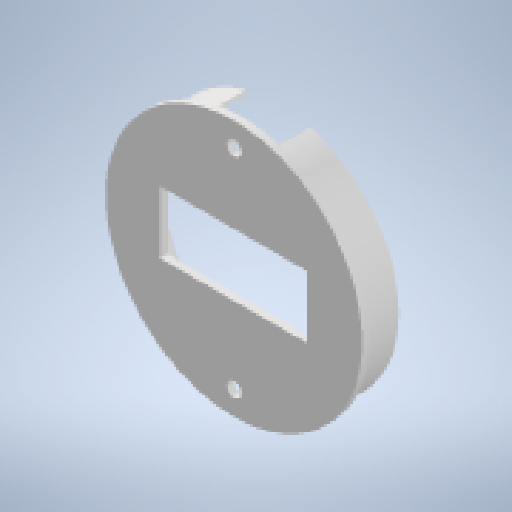
# Autodesk Inventor part: lid2
Saved by Autodesk Inventor 2025.3 (Build 293356000, 356)
## iProperties
Created: 2025-04-21
Part Number: lid2
Material: Generic
Document SubType Name: Modeling
Designer: Owner
Density: 1 g/cm^3
Appearance: Default
Author: Owner
Autodesk Inventor part; units mm, degrees
ref_plane "YZ Plane" through (0, 0, 0) normal (1, 0, 0) x (0, 1, 0)
ref_plane "XZ Plane" through (0, 0, 0) normal (0, 1, 0) x (-1, 0, 0)
ref_plane "XY Plane" through (0, 0, 0) normal (0, 0, 1) x (1, 0, 0)
sketch "Sketch1" plane through (0, 0, 0) normal (0, 0, 1) x (1, 0, 0)
  arc A0 (8.8357, -55.2951) -> (8.8357, 8.2951) centre (0, -23.5) ccw projected
  arc A1 (-8.8357, 8.2951) -> (-8.8357, -55.2951) centre (0, -23.5) ccw projected
  arc A2 (-8.568, 7.3316) -> (-8.568, -54.3316) centre (0, -23.5) ccw
  arc A3 (8.568, -54.3316) -> (8.568, 7.3316) centre (0, -23.5) ccw
  line L0 (8.8357, 8.2951) -> (8.568, 7.3316)
  line L1 (-8.568, 7.3316) -> (-8.8357, 8.2951)
  line L2 (-8.568, -54.3316) -> (-8.8357, -55.2951)
  line L3 (8.568, -54.3316) -> (8.8357, -55.2951)
  point P0 (8.568, 7.3316)
  dimension "d36" = 1
  dimension "d37" = 1
  constraints: 8 end point, 5 point on circle, 2 centre point
  measures "d36" radial gap between concentric circles of A1 A2
  measures "d37" radial gap between concentric circles of A0 A3
extrude "Extrusion1" add sketch "Sketch1" against normal blind 10
ref_plane "Work Plane1" through (0, 0, 0) normal (0, 0, 1) x (1, 0, 0)
sketch "Sketch2" plane through (0, 0, 0) normal (0, 0, 1) x (1, 0, 0)
  circle A0 centre (0, -23.5) radius 35 projected
  circle A1 centre (0, 5) radius 1.5 projected
  circle A2 centre (0, -52) radius 1.5 projected
  circle A3 centre (0, 5) radius 2
  circle A4 centre (0, -52) radius 2
  line L0 (22.5, -34.1118) -> (22.5, -14.1118)
  line L1 (22.5, -14.1118) -> (-22.5, -14.1118)
  line L2 (-22.5, -14.1118) -> (-22.5, -34.1118)
  line L3 (-22.5, -34.1118) -> (22.5, -34.1118)
  line L4 (-16.9429, -31.642) -> (-22.5, -34.1118) construction
  line L5 (-16.9429, -16.5816) -> (-22.5, -14.1118) construction
  line L6 (-20.1463, -14.1118) -> (19.8537, -14.1118)
  line L7 (19.8537, -14.1118) -> (19.8537, -31.1118)
  line L8 (19.8537, -31.1118) -> (-20.1463, -31.1118)
  line L9 (-20.1463, -31.1118) -> (-20.1463, -14.1118)
  point P0 (0, 0)
  point P1 (-8.0435, -8.3885)
  dimension "d4" = 4
  dimension "d5" = 4
  dimension "d6" = 20
  dimension "d7" = 45
  dimension "d32" = 17
  dimension "d33" = 40
  constraints: 20 end point, 4 parallel, 2 centre point, 2 coincident, 2 perpendicular, 2 point on line
  measures "d4" diameter of A3
  measures "d5" diameter of A4
  measures "d6" distance of L3.start L1.end
  measures "d7" distance of L1.end L1.start
  measures "d32" distance of L6.end L7.end
  measures "d33" distance of L6.start L6.end
extrude "Extrusion2" add sketch "Sketch2" along normal blind 2 contours A0 | L3 L2 L1 L9 L8 L7 L0
body "Solid1"
